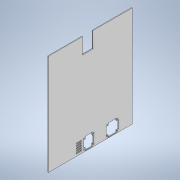
# Autodesk Inventor part: 220310 Left Side
Saved by Autodesk Inventor 2022 (Build 260153000, 153)
## iProperties
Created: 2022-03-10
Part Number: 220310 Left Side
Material: Generic
Document SubType Name: Modeling
Designer: josephinew
Density: 1 g/cm^3
Appearance: Default
Author: josephinew
Autodesk Inventor part; units mm, degrees
ref_plane "YZ Plane" through (0, 0, 0) normal (1, 0, 0) x (0, 1, 0)
ref_plane "XZ Plane" through (0, 0, 0) normal (0, 1, 0) x (-1, 0, 0)
ref_plane "XY Plane" through (0, 0, 0) normal (0, 0, 1) x (1, 0, 0)
sketch "Sketch1" plane through (0, 0, 0) normal (1, 0, 0) x (0, 1, 0)
  line L0 (0, 0) -> (488.95, 0)
  line L1 (488.95, -406.4) -> (0, -406.4)
  line L2 (0, -406.4) -> (0, 0)
  line L3 (488.95, 0) -> (488.95, -165.1)
  line L4 (488.95, -165.1) -> (412.75, -165.1)
  line L5 (412.75, -165.1) -> (412.75, -215.9)
  line L6 (412.75, -215.9) -> (488.95, -215.9)
  line L7 (488.95, 0) -> (488.95, -165.1)
  line L8 (488.95, -215.9) -> (488.95, -406.4)
  line L9 (346.075, 3.175) -> (342.9, 3.175)
  line L10 (342.9, 3.175) -> (346.075, 3.175)
  line L11 (358.775, 3.175) -> (361.95, 3.175)
  line L12 (374.65, 3.175) -> (377.825, 3.175)
  line L13 (390.525, 3.175) -> (393.7, 3.175)
  line L14 (98.425, -406.4) -> (3.175, -406.4)
  line L15 (457.2, 0) -> (0, 0)
  line L16 (3.175, 0) -> (98.425, 0)
  line L17 (0, -406.4) -> (3.175, -406.4)
  dimension "d9" = 3.175
  constraints: 36 end point, 6 perpendicular, 4 parallel, 1 horizontal, 1 point on line
  measures "d9" distance of L1.end L17.end
extrude "Extrusion1" add sketch "Sketch1" along normal blind 3.175
sketch "Sketch2" plane through (0, 0, 0) normal (-1, 0, 0) x (0, 0, 1)
  line L0 (-406.4, 0) -> (-406.4, 488.95) projected
  line L1 (0, 0) -> (-406.4, 0) projected
  line L2 (0, 488.95) -> (0, 0) projected
  line L3 (-165.1, 488.95) -> (0, 488.95) projected
  line L4 (-165.1, 412.75) -> (-165.1, 488.95) projected
  line L5 (-215.9, 412.75) -> (-165.1, 412.75) projected
  line L6 (-215.9, 488.95) -> (-215.9, 412.75) projected
  line L7 (-406.4, 488.95) -> (-215.9, 488.95) projected
  line L8 (-339.725, 53.1114) -> (-339.725, 13.1826)
  line L9 (-279.781, 13.1826) -> (-279.781, 53.1114)
  line L10 (-289.7886, 63.119) -> (-329.7174, 63.119)
  circle A0 centre (-334.7212, 58.1152) radius 2.159
  circle A1 centre (-284.7848, 58.1152) radius 2.159
  circle A2 centre (-334.7212, 8.1788) radius 2.159
  circle A3 centre (-284.7848, 8.1788) radius 2.159
  line L11 (-329.7174, 63.119) -> (-329.7174, 53.1114)
  line L12 (-329.7174, 53.1114) -> (-339.725, 53.1114)
  line L13 (-289.7886, 63.119) -> (-289.7886, 53.1114)
  line L14 (-289.7886, 53.1114) -> (-279.781, 53.1114)
  line L15 (-329.7174, 3.175) -> (-329.7174, 13.1826)
  line L16 (-329.7174, 13.1826) -> (-339.725, 13.1826)
  line L17 (-289.7886, 3.175) -> (-289.7886, 13.1826)
  line L18 (-289.7886, 13.1826) -> (-279.781, 13.1826)
  line L19 (-212.725, 63.1698) -> (-178.2826, 63.1698)
  circle A4 centre (-219.3036, 56.7436) radius 2.54
  circle A5 centre (-219.3036, 9.6012) radius 2.54
  circle A6 centre (-172.1612, 56.7436) radius 2.54
  circle A7 centre (-172.1612, 9.6012) radius 2.54
  line L20 (-136.9822, 10.6172) -> (-158.4706, 10.6172)
  line L21 (-158.4706, 15.6972) -> (-136.9822, 15.6972)
  arc A8 (-136.9822, 10.6172) -> (-136.9822, 15.6972) centre (-136.9822, 13.1572) ccw
  arc A9 (-158.4706, 15.6972) -> (-158.4706, 10.6172) centre (-158.4706, 13.1572) ccw
  line L22 (-136.9822, 20.5994) -> (-158.4706, 20.5994)
  line L23 (-158.4706, 25.6794) -> (-136.9822, 25.6794)
  arc A10 (-136.9822, 20.5994) -> (-136.9822, 25.6794) centre (-136.9822, 23.1394) ccw
  arc A11 (-158.4706, 25.6794) -> (-158.4706, 20.5994) centre (-158.4706, 23.1394) ccw
  line L24 (-136.9822, 30.5816) -> (-158.4706, 30.5816)
  line L25 (-158.4706, 35.6616) -> (-136.9822, 35.6616)
  arc A12 (-136.9822, 30.5816) -> (-136.9822, 35.6616) centre (-136.9822, 33.1216) ccw
  arc A13 (-158.4706, 35.6616) -> (-158.4706, 30.5816) centre (-158.4706, 33.1216) ccw
  line L26 (-136.9822, 40.5638) -> (-158.4706, 40.5638)
  line L27 (-158.4706, 45.6438) -> (-136.9822, 45.6438)
  arc A14 (-136.9822, 40.5638) -> (-136.9822, 45.6438) centre (-136.9822, 43.1038) ccw
  arc A15 (-158.4706, 45.6438) -> (-158.4706, 40.5638) centre (-158.4706, 43.1038) ccw
  line L28 (-136.9822, 50.546) -> (-158.4706, 50.546)
  line L29 (-158.4706, 55.626) -> (-136.9822, 55.626)
  arc A16 (-136.9822, 50.546) -> (-136.9822, 55.626) centre (-136.9822, 53.086) ccw
  arc A17 (-158.4706, 55.626) -> (-158.4706, 50.546) centre (-158.4706, 53.086) ccw
  line L30 (-212.725, 63.1698) -> (-212.725, 50.4698)
  line L31 (-212.725, 50.4698) -> (-219.3036, 50.4698)
  line L32 (-172.1612, 50.4698) -> (-178.2826, 50.4698)
  line L33 (-178.2826, 50.4698) -> (-178.2826, 63.1698)
  line L34 (-178.2826, 3.3274) -> (-178.2826, 16.0274)
  line L35 (-178.2826, 16.0274) -> (-172.1612, 16.0274)
  line L36 (-219.3036, 16.0274) -> (-212.725, 16.0274)
  line L37 (-212.725, 16.0274) -> (-212.725, 3.3274)
  line L38 (-219.3036, 50.4698) -> (-219.3036, 16.0274)
  line L39 (-172.1612, 50.4698) -> (-172.1612, 16.0274)
  line L40 (-403.225, 3.175) -> (-339.725, 3.175)
  line L41 (-329.7174, 3.175) -> (-289.7886, 3.175)
  line L42 (53.975, 3.175) -> (-403.225, 3.175)
  line L43 (-178.2826, 6.0198) -> (-178.2826, 0)
  line L44 (-178.2826, 0) -> (-212.725, 0)
  line L45 (-212.725, 0) -> (-212.725, 6.0198)
  line L46 (-406.4, 0) -> (-406.4, 488.95) projected
  line L47 (-406.4, 0) -> (-406.4, 3.175)
  line L48 (-406.4, 0) -> (-403.225, 0)
  line L49 (-403.225, 0) -> (-403.225, 3.175)
  line L50 (-403.225, 3.175) -> (-406.4, 3.175)
  line L51 (-406.4, 3.175) -> (-406.4, 0)
  point P0 (-332.8924, 0)
  point P1 (-292.9636, 0)
  point P2 (-212.725, 0)
  point P3 (-178.2826, 0)
  point P4 (-212.725, 3.175)
  point P5 (-178.2826, 3.175)
  dimension "d12" = 3.175
  dimension "d15" = 3.175
  dimension "d16" = 3.175
  constraints: 86 end point, 20 point on circle, 18 centre point, 3 parallel, 1 collinear, 1 horizontal, 1 perpendicular, 1 point on line, 2 other
  measures "d12" distance of L0.start L47.end
  measures "d15" distance of L50.end L49.end
  measures "d16" distance of L49.end L48.end
extrude "Extrusion3" cut sketch "Sketch2" against normal blind 25.4 contours L45 L37 L36 L38 L31 L30 L19 L33 L32 L39 L35 L34 L43 L42 | L15 L16 L8 L12 L11 L10 L13 L14 L9 L18 L17 L41 | A0 | A1 | A2 | A3 | A4 | A5 | A6 | A7 | L20 A9 L21 A8 | L22 A11 L23 A10 | L24 A13 L25 A12 | L26 A15 L27 A14 | L28 A17 L29 A16
body "Solid1"
